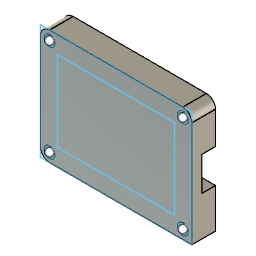
bottom_case (Autodesk Fusion 360 design; units mm, degrees)
Autodesk Fusion 360 part; units mm, degrees
sketch "Sketch1" plane through (0, 0, 0) normal (0, 1, 0) x (1, 0, 0)
  line L0 (-102.9234, -55.5196) -> (-38.7234, -55.5196)
  line L1 (-38.7234, -55.5196) -> (-38.7234, -11.4886)
  line L2 (-38.7234, -11.4886) -> (-102.9234, -11.4886)
  line L3 (-102.9234, -11.4886) -> (-102.9234, -55.5196)
  line L4 (-112.4234, -65.0196) -> (-29.2234, -65.0196)
  line L5 (-29.2234, -65.0196) -> (-29.2234, -1.9886)
  line L6 (-29.2234, -1.9886) -> (-112.4234, -1.9886)
  line L7 (-112.4234, -1.9886) -> (-112.4234, -65.0196)
  circle A0 centre (-107.4234, -60.0196) radius 1.7
  circle A1 centre (-34.2234, -60.0196) radius 1.7
  circle A2 centre (-107.4234, -6.9886) radius 1.7
  circle A3 centre (-34.2234, -6.9886) radius 1.7
  circle A4 centre (-107.4234, -60.0196) radius 3
  circle A5 centre (-107.4234, -6.9886) radius 3
  circle A6 centre (-34.2234, -6.9886) radius 3
  circle A7 centre (-34.2234, -60.0196) radius 3
  dimension "d1" = 64.2
  dimension "d2" = 44.031
  dimension "d3" = 83.2
  dimension "d4" = 63.031
  dimension "d5" = 9.5
  dimension "d6" = 9.5
  dimension "d7" = 3.4
  dimension "d8" = 3.4
  dimension "d9" = 3.4
  dimension "d10" = 3.4
  dimension "d11" = 5
  dimension "d12" = 5
  dimension "d13" = 5
  dimension "d14" = 5
  dimension "d15" = 5
  dimension "d16" = 5
  dimension "d17" = 5
  dimension "d18" = 5
  dimension "d19" = 6
  dimension "d20" = 6
  dimension "d21" = 6
  dimension "d22" = 6
  constraint horizontal L0
  constraint vertical L1
  constraint horizontal L2
  constraint vertical L3
  constraint horizontal L4
  constraint vertical L5
  constraint horizontal L6
  constraint vertical L7
  constraint concentric A0 A4
  constraint concentric A2 A5
  constraint concentric A3 A6
  constraint concentric A1 A7
  measures "d1" distance of L0.start L0.end
  measures "d2" distance of L0.start L2.end
  measures "d3" distance of L4.start L4.end
  measures "d4" distance of L4.start L6.end
  measures "d5" distance of L0 L4
  measures "d6" distance of L1 L5
  measures "d7" diameter of A0
  measures "d8" diameter of A1
  measures "d9" diameter of A2
  measures "d10" diameter of A3
  measures "d11" distance of L7 A2.centre
  measures "d12" distance of L6 A2.centre
  measures "d13" distance of L6 A3.centre
  measures "d14" distance of L5 A3.centre
  measures "d15" distance of L4 A1.centre
  measures "d16" distance of L5 A1.centre
  measures "d17" distance of L4 A0.centre
  measures "d18" distance of L7 A0.centre
  measures "d19" diameter of A4
  measures "d20" diameter of A5
  measures "d21" diameter of A6
  measures "d22" diameter of A7
extrude "Extrude1" add sketch "Sketch1" along normal blind 9.9 from surface at 3.1 contours A4 | A5 | A6 | A7 makes body 1 at (-37.2197, 9.7, 60.1692) makes body 2 at (-31.2271, 9.7, 7.1382) makes body 3 at (-109.5181, 9.7, 62.1672) makes body 4 at (-104.4271, 9.7, 7.1382)
extrude "Extrude2" add sketch "Sketch1" along normal blind 13 contours L4 L5 L6 L7 bodies 1 2 3 4
extrude "Extrude3" add sketch "Sketch1" along normal blind 3 contours L0 L1 L2 L3 bodies 1
sketch "Sketch2" plane through (0, 13, 0) normal (0, 1, 0) x (-1, 0, 0)
  circle A0 centre (34.2234, 60.0196) radius 1.7
  circle A1 centre (107.4234, 6.9886) radius 1.7
  line L0 (102.9234, 55.5196) -> (102.9234, 11.4886)
  line L1 (102.9234, 11.4886) -> (38.7234, 11.4886)
  line L2 (38.7234, 11.4886) -> (38.7234, 55.5196)
  line L3 (38.7234, 55.5196) -> (102.9234, 55.5196)
  line L4 (112.4234, 1.9886) -> (112.4234, 65.0196)
  line L5 (112.4234, 65.0196) -> (29.2234, 65.0196)
  line L6 (29.2234, 65.0196) -> (29.2234, 1.9886)
  line L7 (29.2234, 1.9886) -> (112.4234, 1.9886)
  circle A2 centre (34.2234, 6.9886) radius 1.7
  circle A3 centre (107.4234, 60.0196) radius 1.7
  line L8 (29.2234, 23.7386) -> (38.7234, 23.7386)
  line L9 (38.7234, 23.7386) -> (38.7234, 42.2386)
  line L10 (38.7234, 42.2386) -> (29.2234, 42.2386)
  line L11 (29.2234, 42.2386) -> (29.2234, 23.7386)
  line L12 (29.2234, 1.9886) -> (112.4234, 1.9886)
  dimension "d30" = 18.5
  dimension "d31" = 21.75
  constraint horizontal L8
  constraint vertical L9
  constraint horizontal L10
  constraint vertical L11
  constraint coincident L6 L8.start
  measures "d30" distance of L8.start L10.end
  measures "d31" distance of L8 L12
extrude "Extrude4" cut sketch "Sketch2" against normal blind 7.5 contours L2 L6 L8 L9 L10 L11 bodies 1
fillet "Fillet1" radius 5 1 edges at (-112.4234, 6.5, 65.0196) on bodies 1
fillet "Fillet2" radius 5 1 edges at (-112.4234, 6.5, 1.9886) on bodies 1
fillet "Fillet3" radius 5 1 edges at (-29.2234, 6.5, 65.0196) on bodies 1
